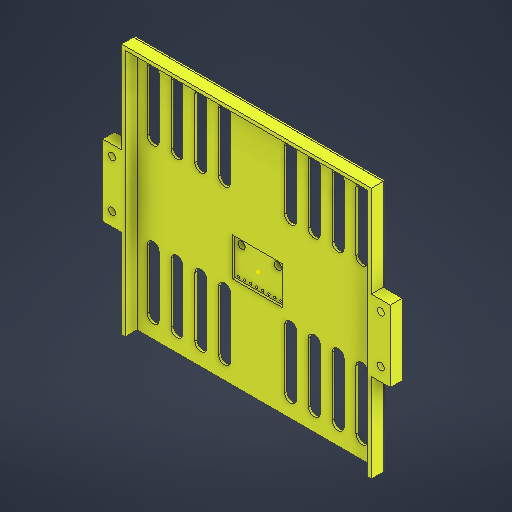
# Autodesk Inventor part: imuholder
Saved by Autodesk Inventor 2027 (Build 310192000, 192)
## iProperties
Created: 2026-06-30
Part Number: imuholder
Material: Generic
Document SubType Name: Modeling
Designer: uchiha
Density: 1 g/cm^3
Appearance: Default
Author: uchiha
Autodesk Inventor part; units mm, degrees
ref_plane "YZ Plane" through (0, 0, 0) normal (1, 0, 0) x (0, 1, 0)
ref_plane "XZ Plane" through (0, 0, 0) normal (0, 1, 0) x (-1, 0, 0)
sketch "Sketch1" plane through (0, 0, 0) normal (0, 0, 1) x (1, 0, 0)
  line L0 (10.4556, 8.1109) -> (10.4556, -7.8891)
  line L1 (-10.5444, 8.1109) -> (10.4556, 8.1109)
  line L2 (-10.5444, -7.8891) -> (-10.5444, 8.1109)
  line L3 (10.4556, -7.8891) -> (-10.5444, -7.8891)
  circle A0 centre (-7.6644, 5.3109) radius 1.5
  circle A1 centre (7.5756, 5.3109) radius 1.5
  circle A2 centre (-8.9344, -6.7891) radius 0.5
  circle A3 centre (-6.3944, -6.7891) radius 0.5
  circle A4 centre (-3.8544, -6.7891) radius 0.5
  circle A5 centre (-1.3144, -6.7891) radius 0.5
  circle A6 centre (1.2256, -6.7891) radius 0.5
  circle A7 centre (3.7656, -6.7891) radius 0.5
  circle A8 centre (6.3056, -6.7891) radius 0.5
  circle A9 centre (8.8456, -6.7891) radius 0.5
  line L4 (12.4556, -9.8891) -> (12.4556, 10.1109)
  line L5 (12.4556, 10.1109) -> (-12.5444, 10.1109)
  line L6 (-12.5444, 10.1109) -> (-12.5444, -9.8891)
  line L7 (-12.5444, -9.8891) -> (12.4556, -9.8891)
  circle A10 centre (7.5756, 5.3109) radius 1.5
  circle A11 centre (-7.6644, 5.3109) radius 1.5
  point P0 (0, 0)
  point P1 (-0.0444, 0.1109)
  dimension "d0" = 2
  dimension "d1" = 15.24
  constraints: 16 end point, 12 centre point, 2 coincident, 2 concentric, 3 other
  measures "d0" distance between parallel lines of L0 L4
  measures "d1" distance of A0.centre A1.centre
extrude "Extrusion1" add sketch "Sketch1" against normal blind 2 contours L0 L3 L2 L1
extrude "Extrusion2" add sketch "Sketch1" along normal blind 1 contours L7 L6 L5 L4
sketch "Sketch2" plane through (0, 0, 0) normal (0, 0, 1) x (1, 0, 0)
  line L0 (12.4556, 10.1109) -> (-12.5444, 10.1109) projected
  line L1 (-12.5444, 10.1109) -> (-12.5444, -9.8891) projected
  line L2 (-12.5444, -9.8891) -> (12.4556, -9.8891) projected
  line L3 (12.4556, -9.8891) -> (12.4556, 10.1109) projected
  line L4 (52.5, -59) -> (-52.5, -59)
  line L5 (-52.5, -59) -> (-52.5, 59)
  line L6 (-52.5, 59) -> (52.5, 59)
  line L7 (52.5, 59) -> (52.5, -59)
  line L8 (52.5, -59) -> (-52.5, 59) construction
  line L9 (-52.5, -59) -> (52.5, 59) construction
  point P0 (0, 0)
  dimension "d6" = 118
  dimension "d7" = 105
  constraints: 12 end point, 2 midpoint, 2 parallel, 1 horizontal, 1 perpendicular
  measures "d6" distance of L6.end L4.start
  measures "d7" distance of L5.end L6.end
extrude "Extrusion3" add sketch "Sketch2" along normal blind 1
sketch "Sketch7" plane through (0, 0, 1) normal (0, 0, 1) x (1, 0, 0)
  point P0 (0, 0)
sketch "Sketch8" plane through (0, 0, 1) normal (0, 0, 1) x (1, 0, 0)
  point P0 (0, 0)
sketch "Sketch9" plane through (0, 0, 1) normal (0, 0, 1) x (1, 0, 0)
  line L0 (43.875, 51.5) -> (43.875, 26.5) construction
  line L1 (46.375, 51.5) -> (46.375, 26.5)
  line L2 (41.375, 26.5) -> (41.375, 51.5)
  arc A0 (46.375, 51.5) -> (41.375, 51.5) centre (43.875, 51.5) ccw
  arc A1 (41.375, 26.5) -> (46.375, 26.5) centre (43.875, 26.5) ccw
  line L3 (52.5, 69) -> (-52.5, 69)
  line L4 (52.5, 69) -> (52.5, -49.0201)
  line L5 (36.375, 51.5) -> (36.375, 26.5)
  arc A2 (36.375, 51.5) -> (31.375, 51.5) centre (33.875, 51.5) ccw
  line L6 (31.375, 26.5) -> (31.375, 51.5)
  arc A3 (31.375, 26.5) -> (36.375, 26.5) centre (33.875, 26.5) ccw
  line L7 (33.875, 51.5) -> (33.875, 26.5) construction
  line L8 (26.375, 51.5) -> (26.375, 26.5)
  arc A4 (26.375, 51.5) -> (21.375, 51.5) centre (23.875, 51.5) ccw
  line L9 (21.375, 26.5) -> (21.375, 51.5)
  arc A5 (21.375, 26.5) -> (26.375, 26.5) centre (23.875, 26.5) ccw
  line L10 (23.875, 51.5) -> (23.875, 26.5) construction
  line L11 (16.375, 51.5) -> (16.375, 26.5)
  arc A6 (16.375, 51.5) -> (11.375, 51.5) centre (13.875, 51.5) ccw
  line L12 (11.375, 26.5) -> (11.375, 51.5)
  arc A7 (11.375, 26.5) -> (16.375, 26.5) centre (13.875, 26.5) ccw
  line L13 (13.875, 51.5) -> (13.875, 26.5) construction
  line L14 (46.375, -13.5) -> (46.375, -38.5)
  arc A8 (46.375, -13.5) -> (41.375, -13.5) centre (43.875, -13.5) ccw
  line L15 (41.375, -38.5) -> (41.375, -13.5)
  arc A9 (41.375, -38.5) -> (46.375, -38.5) centre (43.875, -38.5) ccw
  line L16 (43.875, -13.5) -> (43.875, -38.5) construction
  line L17 (36.375, -13.5) -> (36.375, -38.5)
  arc A10 (36.375, -13.5) -> (31.375, -13.5) centre (33.875, -13.5) ccw
  line L18 (31.375, -38.5) -> (31.375, -13.5)
  arc A11 (31.375, -38.5) -> (36.375, -38.5) centre (33.875, -38.5) ccw
  line L19 (33.875, -13.5) -> (33.875, -38.5) construction
  line L20 (26.375, -13.5) -> (26.375, -38.5)
  arc A12 (26.375, -13.5) -> (21.375, -13.5) centre (23.875, -13.5) ccw
  line L21 (21.375, -38.5) -> (21.375, -13.5)
  arc A13 (21.375, -38.5) -> (26.375, -38.5) centre (23.875, -38.5) ccw
  line L22 (23.875, -13.5) -> (23.875, -38.5) construction
  line L23 (16.375, -13.5) -> (16.375, -38.5)
  arc A14 (16.375, -13.5) -> (11.375, -13.5) centre (13.875, -13.5) ccw
  line L24 (11.375, -38.5) -> (11.375, -13.5)
  arc A15 (11.375, -38.5) -> (16.375, -38.5) centre (13.875, -38.5) ccw
  line L25 (13.875, -13.5) -> (13.875, -38.5) construction
  line L26 (0, 69) -> (0, -59)
  line L27 (-52.5, -59) -> (52.5, -59) projected
  line L28 (-43.875, 51.5) -> (-43.875, 26.5) construction
  line L29 (-46.375, 51.5) -> (-46.375, 26.5)
  line L30 (-41.375, 26.5) -> (-41.375, 51.5)
  arc A16 (-41.375, 51.5) -> (-46.375, 51.5) centre (-43.875, 51.5) ccw
  arc A17 (-46.375, 26.5) -> (-41.375, 26.5) centre (-43.875, 26.5) ccw
  line L31 (-36.375, 51.5) -> (-36.375, 26.5)
  arc A18 (-31.375, 51.5) -> (-36.375, 51.5) centre (-33.875, 51.5) ccw
  line L32 (-31.375, 26.5) -> (-31.375, 51.5)
  arc A19 (-36.375, 26.5) -> (-31.375, 26.5) centre (-33.875, 26.5) ccw
  line L33 (-33.875, 51.5) -> (-33.875, 26.5) construction
  line L34 (-26.375, 51.5) -> (-26.375, 26.5)
  arc A20 (-21.375, 51.5) -> (-26.375, 51.5) centre (-23.875, 51.5) ccw
  line L35 (-21.375, 26.5) -> (-21.375, 51.5)
  arc A21 (-26.375, 26.5) -> (-21.375, 26.5) centre (-23.875, 26.5) ccw
  line L36 (-23.875, 51.5) -> (-23.875, 26.5) construction
  line L37 (-16.375, 51.5) -> (-16.375, 26.5)
  arc A22 (-11.375, 51.5) -> (-16.375, 51.5) centre (-13.875, 51.5) ccw
  line L38 (-11.375, 26.5) -> (-11.375, 51.5)
  arc A23 (-16.375, 26.5) -> (-11.375, 26.5) centre (-13.875, 26.5) ccw
  line L39 (-13.875, 51.5) -> (-13.875, 26.5) construction
  line L40 (-46.375, -13.5) -> (-46.375, -38.5)
  arc A24 (-41.375, -13.5) -> (-46.375, -13.5) centre (-43.875, -13.5) ccw
  line L41 (-41.375, -38.5) -> (-41.375, -13.5)
  arc A25 (-46.375, -38.5) -> (-41.375, -38.5) centre (-43.875, -38.5) ccw
  line L42 (-43.875, -13.5) -> (-43.875, -38.5) construction
  line L43 (-36.375, -13.5) -> (-36.375, -38.5)
  arc A26 (-31.375, -13.5) -> (-36.375, -13.5) centre (-33.875, -13.5) ccw
  line L44 (-31.375, -38.5) -> (-31.375, -13.5)
  arc A27 (-36.375, -38.5) -> (-31.375, -38.5) centre (-33.875, -38.5) ccw
  line L45 (-33.875, -13.5) -> (-33.875, -38.5) construction
  line L46 (-26.375, -13.5) -> (-26.375, -38.5)
  arc A28 (-21.375, -13.5) -> (-26.375, -13.5) centre (-23.875, -13.5) ccw
  line L47 (-21.375, -38.5) -> (-21.375, -13.5)
  arc A29 (-26.375, -38.5) -> (-21.375, -38.5) centre (-23.875, -38.5) ccw
  line L48 (-23.875, -13.5) -> (-23.875, -38.5) construction
  line L49 (-16.375, -13.5) -> (-16.375, -38.5)
  arc A30 (-11.375, -13.5) -> (-16.375, -13.5) centre (-13.875, -13.5) ccw
  line L50 (-11.375, -38.5) -> (-11.375, -13.5)
  arc A31 (-16.375, -38.5) -> (-11.375, -38.5) centre (-13.875, -38.5) ccw
  line L51 (-13.875, -13.5) -> (-13.875, -38.5) construction
  line L52 (52.5, 59) -> (-52.5, 59) projected
  point P0 (0, 0)
  point P1 (43.875, 39)
  point P2 (33.875, 39)
  point P3 (23.875, 39)
  point P4 (13.875, 39)
  point P5 (43.875, -26)
  point P6 (33.875, -26)
  point P7 (23.875, -26)
  point P8 (13.875, -26)
  point P9 (-43.875, 39)
  point P10 (-33.875, 39)
  point P11 (-23.875, 39)
  point P12 (-13.875, 39)
  point P13 (-43.875, -26)
  point P14 (-33.875, -26)
  point P15 (-23.875, -26)
  point P16 (-13.875, -26)
  point P17 (33.875, 39)
  dimension "d23" = 5
  dimension "d25" = 25
  dimension "d28" = 10
  dimension "d31" = 65
  dimension "d46" = 20
  constraints: 134 end point, 64 point on circle, 56 symmetric about line, 32 centre point, 4 midpoint, 4 tangent, 3 vertical, 1 horizontal, 1 parallel, 100 other
  measures "d23" distance between parallel lines of L2 L1
  measures "d25" distance of L1.start L1.end
  measures "d28" distance of L1.start L5.start
  measures "d31" distance of L1.start L14.start
  measures "d46" distance from line of point (33.875, 39) L52
extrude "Extrusion9" cut sketch "Sketch9" against normal blind 2 contours L1 A1 L2 A0 | L5 A3 L6 A2 | L8 A5 L9 A4 | L11 A7 L12 A6 | L14 A9 L15 A8 | L17 A11 L18 A10 | L20 A13 L21 A12 | L23 A15 L24 A14 | A16 L30 A17 L29 | A18 L32 A19 L31 | A20 L35 A21 L34 | A22 L38 A23 L37 | A24 L41 A25 L40 | A26 L44 A27 L43 | A28 L47 A29 L46 | A30 L50 A31 L49
sketch "Sketch10" plane through (0, 0, 1) normal (0, 0, 1) x (1, 0, 0)
  circle A0 centre (56.8501, -3.632) radius 1.5
  circle A1 centre (-56.1499, 16.368) radius 1.5
  circle A2 centre (56.8501, 16.368) radius 1.5
  circle A3 centre (-56.1499, -3.632) radius 1.5
  line L0 (52.8501, 59.2753) -> (52.8501, 20.7377)
  line L1 (-52.1499, 59.2753) -> (52.8501, 59.2753)
  line L2 (-52.1499, 20.7377) -> (-52.1499, 59.2753)
  line L3 (-52.1499, 20.7377) -> (-60.1499, 20.7377)
  line L4 (-60.1499, 20.7377) -> (-60.1499, -9.2623)
  line L5 (-60.1499, -9.2623) -> (-52.1499, -9.2623)
  line L6 (-52.1499, -58.7248) -> (-52.1499, -9.2623)
  line L7 (52.8501, -58.7248) -> (-52.1499, -58.7248)
  line L8 (52.8501, -9.2623) -> (52.8501, -58.7248)
  line L9 (52.8501, -9.2623) -> (60.8501, -9.2623)
  line L10 (60.8501, -9.2623) -> (60.8501, 20.7377)
  line L11 (60.8501, 20.7377) -> (52.8501, 20.7377)
  line L12 (51.3501, -57.2248) -> (51.3501, 57.7753)
  line L13 (-50.6499, -57.2248) -> (51.3501, -57.2248)
  line L14 (-50.6499, 57.7753) -> (-50.6499, -57.2248)
  line L15 (51.3501, 57.7753) -> (-50.6499, 57.7753)
  line L16 (60.8774, 20.7651) -> (60.8774, -9.2896)
  line L17 (60.8774, -9.2896) -> (52.8774, -9.2896)
  line L18 (52.8774, -9.2896) -> (52.8774, -58.7521)
  line L19 (52.8774, -58.7521) -> (-52.1773, -58.7521)
  line L20 (-52.1773, -58.7521) -> (-52.1773, -9.2896)
  line L21 (-52.1773, -9.2896) -> (-60.1773, -9.2896)
  line L22 (-60.1773, -9.2896) -> (-60.1773, 20.7651)
  line L23 (-60.1773, 20.7651) -> (-52.1773, 20.7651)
  line L24 (-52.1773, 20.7651) -> (-52.1773, 59.3026)
  line L25 (-52.1773, 59.3026) -> (52.8774, 59.3026)
  line L26 (52.8774, 59.3026) -> (52.8774, 20.7651)
  line L27 (52.8774, 20.7651) -> (60.8774, 20.7651)
  point P0 (0, 0)
  point P1 (0.3501, 0.2752)
  constraints: 56 end point, 4 centre point, 11 other
extrude "Extrusion10" add sketch "Sketch10" along normal blind 5 contours L0 L11 L10 L9 L8 L7 L6 L5 L4 L3 L2 L1
ref_plane "Work Plane2" through (-82.1499, -58.7248, 1) normal (-1, 0, 0) x (0, 0, 1)
sketch "Sketch11" plane through (-82.1499, -58.7248, 1) normal (-1, 0, 0) x (0, 0, 1)
  line L0 (-1, -0.2752) -> (2.0041, -0.2752)
  line L1 (2.0041, -0.2752) -> (2.0041, 12.1798)
  line L2 (2.0041, 12.1798) -> (-1, 12.1798)
  line L3 (-1, 12.1798) -> (-1, -0.2752)
  line L4 (-1, -0.2752) -> (0, -0.2752) projected
  point P0 (-1, 58.7248)
  dimension "d43" = 12.455
  constraints: 8 end point, 2 parallel, 1 collinear, 1 horizontal, 1 perpendicular
  measures "d43" distance of L2.end L0.start
extrude "Extrusion11" cut sketch "Sketch11" against normal blind 1000
sketch "Sketch12" plane through (-52.1499, -58.7248, 6) normal (-1, 0, 0) x (0, 0, 1)
  line L0 (-2.9959, 12.1798) -> (-5, 12.1798) projected
  line L1 (0, 0) -> (0, 49.4625) projected
  line L2 (-2.9959, 12.1798) -> (0, 12.1798)
  line L3 (0, 12.1798) -> (0, 0)
  line L4 (0, 0) -> (-2.9959, 0)
  line L5 (-2.9959, 0) -> (-2.9959, 12.1798)
  point P0 (-6, 58.7248)
  constraints: 8 end point, 2 parallel, 1 horizontal, 1 perpendicular
extrude "Extrusion12" cut sketch "Sketch12" against normal blind 500
body "Solid1"
